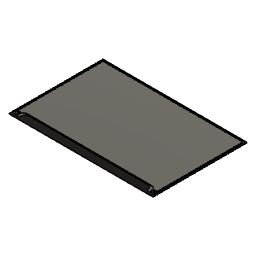
openbook_3d_file_ariton_alexandru (Autodesk Fusion 360 archive; units mm, degrees)
design "Screen"
Autodesk Fusion 360 part; units mm, degrees
sketch "Sketch1" plane through (0, 0, 0) normal (0, 0, 1) x (1, 0, 0)
  line L0 (-75, 50) -> (95.2, 50)
  line L1 (95.2, 50) -> (95.2, -61.2)
  line L2 (95.2, -61.2) -> (-75, -61.2)
  line L3 (-75, -61.2) -> (-75, 50)
  dimension "d1" = 170.2
  dimension "d2" = 111.2
  constraint horizontal L0
  constraint vertical L1
  constraint horizontal L2
  constraint vertical L3
  measures "d1" distance of L0.start L0.end
  measures "d2" distance of L0.start L2.end
extrude "Extrude1" add sketch "Sketch1" along normal blind 1.18 makes body 1
extrude "Extrude2" cut 1 faces at (-18.2667, 12.9333, 1.18) along direction (0, 0, -1) blind 0.48 on bodies 1 bodies 1
sketch "Sketch2" plane through (0, 0, 0.7) normal (0, 0, 1) x (-1, 0, 0)
  line L0 (75, 61.2) -> (-95.2, 61.2)
  line L1 (-95.2, 61.2) -> (-95.2, -50)
  line L2 (-95.2, -50) -> (75, -50)
  line L3 (75, -50) -> (75, 61.2)
  line L4 (150, -120) -> (314.8, -120)
  line L5 (314.8, -120) -> (314.8, -224.09)
  line L6 (314.8, -224.09) -> (150, -224.09)
  line L7 (150, -224.09) -> (150, -120)
  dimension "d7" = 164.8
  dimension "d8" = 104.09
  constraint horizontal L4
  constraint vertical L5
  constraint horizontal L6
  constraint vertical L7
  measures "d7" distance of L4.start L4.end
  measures "d8" distance of L4.start L6.end
extrude "Extrude3" add sketch "Sketch2" along normal blind 0.48 separate body contours L4 L5 L6 L7 makes body 2
move_body "Move1" bodies 2 to x (1, 0, 0) y (0, 1, 0) z (0, 0, 1) at (239.8, 0, 0)
move_body "Move2" bodies 2 to x (1, 0, 0) y (0, 1, 0) z (0, 0, 1) at (2.7, 0, 0)
move_body "Move3" bodies 2 to x (1, 0, 0) y (0, 1, 0) z (0, 0, 1) at (0, -175, 0)
move_body "Move4" bodies 2 to x (1, 0, 0) y (0, 1, 0) z (0, 0, 1) at (0, 0.91, 0)
move_body "Move5" bodies 2 to x (1, 0, 0) y (0, 1, 0) z (0, 0, 1) at (0, -2.7, 0)
move_body "Move6" bodies 2 to x (1, 0, 0) y (0, 1, 0) z (0, 0, 1) at (0, 0, -1.18)
sketch "Sketch3" plane through (0, 0, -0.48) normal (0, 0, -1) x (1, 0, 0)
  line L0 (-72.3, -47.3) -> (92.5, -47.3)
  line L1 (92.5, -47.3) -> (92.5, 56.79)
  line L2 (92.5, 56.79) -> (-72.3, 56.79)
  line L3 (-72.3, 56.79) -> (-72.3, -47.3)
  line L4 (-67.9582, 56.79) -> (88.022, 56.79)
  line L5 (88.022, 56.79) -> (88.022, 50.79)
  line L6 (88.022, 50.79) -> (-67.9582, 50.79)
  line L7 (-67.9582, 50.79) -> (-67.9582, 56.79)
  dimension "d11" = 6
  constraint horizontal L4
  constraint vertical L5
  constraint horizontal L6
  constraint vertical L7
  constraint coincident L2 L4.start
  measures "d11" distance of L4.start L6.end
extrude "Extrude4" cut sketch "Sketch3" against normal blind 0.48 contours L2 L4 L5 L6 L7 bodies 2
fillet "Fillet1" radius 4.75 1 edges at (88.022, -50.79, -0.24) on bodies 2
fillet "Fillet2" radius 4.75 1 edges at (-67.9582, -50.79, -0.24) on bodies 2
move_body "Move7" bodies 2 to x (1, 0, 0) y (0, 1, 0) z (0, 0, 1) at (0, 0, 1.18)
move_body "Move8" bodies 1 2 to x (1, 0, 0) y (0, 1, 0) z (0, 0, 1) at (0, 0, -1.18)
sketch "Sketch4" plane through (0, 0, -1.18) normal (0, 0, -1) x (1, 0, 0)
  line L0 (95.2, 61.2) -> (-75, 61.2)
  line L1 (-75, 61.2) -> (-75, -50)
  line L2 (-75, -50) -> (95.2, -50)
  line L3 (95.2, -50) -> (95.2, 61.2)
  line L4 (90, -165) -> (-73.2, -165)
  line L5 (-73.2, -165) -> (-73.2, -67.08)
  line L6 (-73.2, -67.08) -> (90, -67.08)
  line L7 (90, -67.08) -> (90, -165)
  dimension "d18" = 163.2
  dimension "d19" = 97.92
  constraint horizontal L4
  constraint vertical L5
  constraint horizontal L6
  constraint vertical L7
  measures "d18" distance of L4.start L4.end
  measures "d19" distance of L4.start L6.end
extrude "Extrude5" add sketch "Sketch4" along normal blind 0.2 separate body contours L4 L5 L6 L7 makes body 3
extrude "Extrude6" cut 1 faces at (-18.2667, 12.9333, -1.18) along direction (0, 0, 1) blind 0.2 on bodies 1 bodies 1
move_body "Move9" bodies 3 to x (1, 0, 0) y (0, 1, 0) z (0, 0, 1) at (-1.8, -115, 0)
move_body "Move10" bodies 3 to x (1, 0, 0) y (0, 1, 0) z (0, 0, 1) at (3.5, 0, 0)
move_body "Move11" bodies 3 to x (1, 0, 0) y (0, 1, 0) z (0, 0, 1) at (0, -3.5, 0)
move_body "Move12" bodies 3 to x (1, 0, 0) y (0, 1, 0) z (0, 0, 1) at (0, 0, 0.2)
move_body "Move13" bodies 1 2 3 to x (1, 0, 0) y (0, 1, 0) z (0, 0, 1) at (0, 0, 1)
move_body "Move14" bodies 1 2 3 to x (1, 0, 0) y (0, 1, 0) z (0, 0, 1) at (0, 0, -0.35)
sketch "Sketch5" plane through (0, 0, 0.65) normal (0, 0, 1) x (-1, 0, 0)
  line L0 (67.9582, 56.79) -> (67.9582, 55.54)
  arc A0 (63.2082, 50.79) -> (67.9582, 55.54) centre (63.2082, 55.54) ccw
  line L1 (63.2082, 50.79) -> (-83.272, 50.79)
  arc A1 (-88.022, 55.54) -> (-83.272, 50.79) centre (-83.272, 55.54) ccw
  line L2 (-88.022, 55.54) -> (-88.022, 56.79)
  line L3 (-88.022, 56.79) -> (-92.5, 56.79)
  line L4 (-92.5, 56.79) -> (-92.5, -47.3)
  line L5 (-92.5, -47.3) -> (72.3, -47.3)
  line L6 (72.3, -47.3) -> (72.3, 56.79)
  line L7 (72.3, 56.79) -> (67.9582, 56.79)
  line L8 (-75, 200) -> (92.08, 200)
  line L9 (92.08, 200) -> (92.08, 92.91)
  line L10 (92.08, 92.91) -> (-75, 92.91)
  line L11 (-75, 92.91) -> (-75, 200)
  dimension "d24" = 167.08
  dimension "d25" = 107.09
  constraint horizontal L8
  constraint vertical L9
  constraint horizontal L10
  constraint vertical L11
  measures "d24" distance of L8.start L8.end
  measures "d25" distance of L8.start L10.end
extrude "Extrude7" add sketch "Sketch5" along normal blind 0.2 separate body contours L8 L9 L10 L11 makes body 4
move_body "Move15" bodies 4 to x (1, 0, 0) y (0, 1, 0) z (0, 0, 1) at (17.1, 143.21, 0)
move_body "Move16" bodies 4 to x (1, 0, 0) y (0, 1, 0) z (0, 0, 1) at (1.5, -1.5, 0)
move_body "Move17" bodies 4 to x (1, 0, 0) y (0, 1, 0) z (0, 0, 1) at (0, 0, -0.5)
sketch "Sketch6" plane through (0, 0, 0.65) normal (0, 0, 1) x (-1, 0, 0)
  line L0 (67.9582, 56.79) -> (67.9582, 55.54)
  arc A0 (63.2082, 50.79) -> (67.9582, 55.54) centre (63.2082, 55.54) ccw
  line L1 (63.2082, 50.79) -> (-83.272, 50.79)
  arc A1 (-88.022, 55.54) -> (-83.272, 50.79) centre (-83.272, 55.54) ccw
  line L2 (-88.022, 55.54) -> (-88.022, 56.79)
  line L3 (-88.022, 56.79) -> (-92.5, 56.79)
  line L4 (-92.5, 56.79) -> (-92.5, -47.3)
  line L5 (-92.5, -47.3) -> (72.3, -47.3)
  line L6 (72.3, -47.3) -> (72.3, 56.79)
  line L7 (72.3, 56.79) -> (67.9582, 56.79)
  line L8 (65, 52, -0.28) -> (-85, 52, -0.28)
  line L9 (-85, 52, -0.28) -> (-85, 59, -0.28)
  line L10 (-85, 59, -0.28) -> (65, 59, -0.28)
  line L11 (65, 59, -0.28) -> (65, 52, -0.28)
extrude "Extrude8" cut sketch "Sketch6" against normal blind 0.2 contours L8 L9 L10 L11 in plane through (0, 0, 0.37) normal (0, 0, 1) bodies 4
delete_face "DeleteFace1" 1 faces at (35, -54.0967, 0.17) on bodies 4
fillet "Fillet3" radius 4.95 1 edges at (-65, -52, 0.25) on bodies 4
fillet "Fillet4" radius 4.95 1 edges at (85, -52, 0.25) on bodies 4
sketch "Sketch7" plane through (0, 0, 0.65) normal (0, 0, 1) x (-1, 0, 0)
  line L0 (67.9582, 56.79) -> (67.9582, 55.54)
  arc A0 (63.2082, 50.79) -> (67.9582, 55.54) centre (63.2082, 55.54) ccw
  line L1 (63.2082, 50.79) -> (-83.272, 50.79)
  arc A1 (-88.022, 55.54) -> (-83.272, 50.79) centre (-83.272, 55.54) ccw
  line L2 (-88.022, 55.54) -> (-88.022, 56.79)
  line L3 (-88.022, 56.79) -> (-92.5, 56.79)
  line L4 (-92.5, 56.79) -> (-92.5, -47.3)
  line L5 (-92.5, -47.3) -> (72.3, -47.3)
  line L6 (72.3, -47.3) -> (72.3, 56.79)
  line L7 (72.3, 56.79) -> (67.9582, 56.79)
  circle A2 centre (70, 54) radius 1.2382
extrude "Extrude9" cut sketch "Sketch7" against normal blind 3 contours A2 bodies 1 2 4
sketch "Sketch8" plane through (0, 0, 0.65) normal (0, 0, 1) x (-1, 0, 0)
  circle A0 centre (70, 54) radius 1.2382
  line L0 (67.9582, 56.79) -> (67.9582, 55.54)
  arc A1 (63.2082, 50.79) -> (67.9582, 55.54) centre (63.2082, 55.54) ccw
  line L1 (63.2082, 50.79) -> (-83.272, 50.79)
  arc A2 (-88.022, 55.54) -> (-83.272, 50.79) centre (-83.272, 55.54) ccw
  line L2 (-88.022, 55.54) -> (-88.022, 56.79)
  line L3 (-88.022, 56.79) -> (-92.5, 56.79)
  line L4 (-92.5, 56.79) -> (-92.5, -47.3)
  line L5 (-92.5, -47.3) -> (72.3, -47.3)
  line L6 (72.3, -47.3) -> (72.3, 56.79)
  line L7 (72.3, 56.79) -> (67.9582, 56.79)
  circle A3 centre (-90.3, 54.5) radius 1.1438
extrude "Extrude10" cut sketch "Sketch8" against normal blind 6 contours A3 bodies 1 2 4

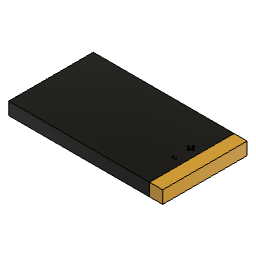
design "Baterie"
Autodesk Fusion 360 part; units mm, degrees
sketch "Sketch1" plane through (0, 0, 0) normal (0, 1, 0) x (1, 0, 0)
  line L0 (-20, -35) -> (22, -35)
  line L1 (22, -35) -> (22, 41.5)
  line L2 (22, 41.5) -> (-20, 41.5)
  line L3 (-20, 41.5) -> (-20, -35)
  dimension "d1" = 42
  dimension "d2" = 76.5
  constraint horizontal L0
  constraint vertical L1
  constraint horizontal L2
  constraint vertical L3
  measures "d1" distance of L0.start L0.end
  measures "d2" distance of L0.start L2.end
extrude "Extrude1" add sketch "Sketch1" along normal blind 6.3 makes body 1
move_body "Move1" bodies 1 to x (0, 1, 0) y (0, 0, 1) z (1, 0, 0) at (-16.75, 23.15, -6.4)
move_body "Move2" bodies 1 to x (1, 0, 0) y (0, 1, 0) z (0, 0, 1) at (20, -25, 0)
copy_body "CopyPasteBodies1" bodies 1 makes body 2
move_body "Move3" bodies 2 to x (1, 0, 0) y (0, 1, 0) z (0, 0, 1) at (0, 45, 0)
extrude "Extrude2" cut 1 faces at (-38.25, 51.15, -4.3) along direction (1, 0, 0) blind 70 on bodies 2 bodies 2
move_face "OffsetFaces1" offset -6.5 1 faces at (38.25, -7.85, -4.3) on bodies 1
move_body "Move4" bodies 2 to x (1, 0, 0) y (0, 1, 0) z (0, 0, 1) at (0, -45, 0)
sketch "Sketch2" plane through (0, 0, 0) normal (0, 0, 1) x (1, 0, 0)
  line L0 (-12, 21) -> (-7, 21) construction
  line L1 (-7, 21) -> (-7, 26) construction
  line L2 (-7, 26) -> (-12, 26) construction
  line L3 (-12, 26) -> (-12, 21) construction
  dimension "d8" = 5
  text T0 "+" font "Arial" height 5 align centre middle in box 5 x 5 at (-12, 21) x (1, 0) y (0, 1) spacing 1 kerned
extrude "Extrude3" add sketch "Sketch2" along normal blind 0.3 separate body text T0 makes body 3
move_body "Move5" bodies 3 to x (1, 0, 0) y (0, 1, 0) z (0, 0, 1) at (37, -19, -0.1)
sketch "Sketch3" plane through (0, 0, 0) normal (0, 0, 1) x (1, 0, 0)
  line L0 (25, -6) -> (29, -6) construction
  line L1 (29, -6) -> (29, -2) construction
  line L2 (29, -2) -> (25, -2) construction
  line L3 (25, -2) -> (25, -6) construction
  dimension "d11" = 5
  text T0 "-" font "Arial" height 5 align centre middle in box 4 x 4 at (25, -6) x (1, 0) y (0, 1) spacing 1 kerned
extrude "Extrude4" add sketch "Sketch3" along normal blind 0.3 separate body text T0 makes body 4
move_body "Move6" bodies 4 to x (1, 0, 0) y (0, 1, 0) z (0, 0, 1) at (0, 0, -0.1)
move_body "Move7" bodies 4 to x (1, 0, 0) y (0, 1, 0) z (0, 0, 1) at (0.5, 0, 0)
move_body "Move8" bodies 3 4 to x (1, 0, 0) y (0, 1, 0) z (0, 0, 1) at (0, -2, 0)
